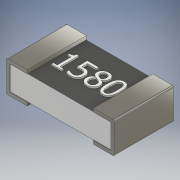
# Autodesk Inventor part: 21-1001
Saved by Autodesk Inventor 2018 (Build 220112000, 112)
## iProperties
Created: 2019-09-21
Part Number: 21-1001
Material: Copper
Document SubType Name: Modeling
Designer: Bradley
Density: 8.94 g/cm^3
Appearance: Smooth - White
Author: Bradley
Autodesk Inventor part; units mm, degrees
ref_plane "YZ Plane" through (0, 0, 0) normal (1, 0, 0) x (0, 1, 0)
ref_plane "XZ Plane" through (0, 0, 0) normal (0, 1, 0) x (-1, 0, 0)
ref_plane "XY Plane" through (0, 0, 0) normal (0, 0, 1) x (1, 0, 0)
sketch "Sketch1" plane through (0, 0, 0) normal (0, 1, 0) x (-1, 0, 0)
  line L0 (0.725, 0.175) -> (-0.725, 0.175)
  line L1 (-0.725, 0.175) -> (-0.725, -0.175)
  line L2 (-0.725, -0.175) -> (0.725, -0.175)
  line L3 (0.725, -0.175) -> (0.725, 0.175)
  line L4 (0.475, 0.175) -> (0.475, 0.225)
  line L5 (0.475, 0.225) -> (0.775, 0.225)
  line L6 (0.775, 0.225) -> (0.775, -0.225)
  line L7 (0.775, -0.225) -> (0.475, -0.225)
  line L8 (0.475, -0.225) -> (0.475, -0.175)
  line L9 (-0.475, 0.175) -> (-0.475, 0.225)
  line L10 (-0.475, 0.225) -> (-0.775, 0.225)
  line L11 (-0.775, 0.225) -> (-0.775, -0.225)
  line L12 (-0.775, -0.225) -> (-0.475, -0.225)
  line L13 (-0.475, -0.175) -> (-0.475, -0.225)
  line L14 (0.475, 0.175) -> (-0.475, 0.175)
  point P0 (0, 0)
  point P1 (0, 0.175)
  point P2 (0.725, 0)
  dimension "d0" = 1.55
  dimension "d1" = 0.05
  dimension "d2" = 0.05
  dimension "d3" = 0.45
  dimension "d4" = 0.3
  constraints: 30 end point, 12 point on line, 7 perpendicular, 3 collinear, 3 midpoint, 2 parallel, 1 horizontal, 1 horizontal alignment, 1 vertical, 1 vertical alignment
  measures "d0" distance between parallel lines of L11 L6
  measures "d1" distance of L7.end L8.end
  measures "d2" distance between parallel lines of L6 L3
  measures "d3" distance of L5.end L6.end
  measures "d4" distance of L6.end L7.end
extrude "Extrusion1" add sketch "Sketch1" along normal mid plane 0.85 contours L0 L4 L5 L6 L7 L8 L2 L3 | L0 L1 L2 L13 L12 L11 L10 L9
extrude "Extrusion2" add sketch "Sketch1" along normal mid plane 0.84 contours L3 L2 L1 L0
sketch "Sketch2" plane through (-0.475, -0.42, 0.175) normal (0, 0, 1) x (1, 0, 0)
  line L0 (0, 0) -> (0, 0.84) projected
  line L1 (0.95, 0) -> (0, 0) projected
  line L2 (0.95, 0) -> (0.95, 0.84) projected
  line L3 (0, 0.84) -> (0.95, 0.84) projected
  line L4 (0, 0.42) -> (0.95, 0.42) construction
  line L5 (0.2166, 0.27) -> (0.0702, 0.27)
  line L6 (0.0702, 0.27) -> (0.0702, 0.3006)
  line L7 (0.0702, 0.3006) -> (0.1247, 0.3006)
  line L8 (0.1247, 0.3006) -> (0.1247, 0.5017)
  line L9 (0.1247, 0.5017) -> (0.0702, 0.5017)
  line L10 (0.0702, 0.5017) -> (0.0702, 0.5292)
  spline S0 degree 2 poles (0.0702, 0.5292) (0.1011, 0.5292) (0.1303, 0.5467) (0.1322, 0.571) knots 0 0 0 1 2 2 2
  line L11 (0.1322, 0.571) -> (0.1633, 0.571)
  line L12 (0.1633, 0.571) -> (0.1633, 0.3006)
  line L13 (0.1633, 0.3006) -> (0.2166, 0.3006)
  line L14 (0.2166, 0.3006) -> (0.2166, 0.27)
  spline S1 degree 2 poles (0.4536, 0.3653) (0.4536, 0.3437) (0.4397, 0.3067) (0.4271, 0.2931) knots 0 0 0 1 2 2 2
  spline S2 degree 2 poles (0.4271, 0.2931) (0.4145, 0.2795) (0.3768, 0.2637) (0.3534, 0.2637) knots 0 0 0 1 2 2 2
  spline S3 degree 2 poles (0.3534, 0.2637) (0.3321, 0.2637) (0.2902, 0.2732) (0.2749, 0.2807) knots 0 0 0 1 2 2 2
  line L15 (0.2749, 0.2807) -> (0.2749, 0.3232)
  line L16 (0.2749, 0.3232) -> (0.2778, 0.3232)
  spline S4 degree 2 poles (0.2778, 0.3232) (0.2825, 0.3198) (0.2997, 0.3111) (0.3102, 0.3072) knots 0 0 0 1 2 2 2
  spline S5 degree 2 poles (0.3102, 0.3072) (0.3221, 0.3031) (0.3418, 0.2984) (0.3542, 0.2984) knots 0 0 0 1 2 2 2
  spline S6 degree 2 poles (0.3542, 0.2984) (0.3663, 0.2984) (0.3892, 0.3072) (0.3974, 0.3167) knots 0 0 0 1 2 2 2
  spline S7 degree 2 poles (0.3974, 0.3167) (0.405, 0.3257) (0.4128, 0.3495) (0.4128, 0.3655) knots 0 0 0 1 2 2 2
  spline S8 degree 2 poles (0.4128, 0.3655) (0.4128, 0.3816) (0.404, 0.402) (0.3957, 0.4088) knots 0 0 0 1 2 2 2
  spline S9 degree 2 poles (0.3957, 0.4088) (0.3872, 0.4164) (0.362, 0.4227) (0.3466, 0.4227) knots 0 0 0 1 2 2 2
  spline S10 degree 2 poles (0.3466, 0.4227) (0.3301, 0.4227) (0.2973, 0.4176) (0.2873, 0.4154) knots 0 0 0 1 2 2 2
  line L17 (0.2873, 0.4154) -> (0.2873, 0.57)
  line L18 (0.2873, 0.57) -> (0.4519, 0.57)
  line L19 (0.4519, 0.57) -> (0.4519, 0.5347)
  line L20 (0.4519, 0.5347) -> (0.326, 0.5347)
  line L21 (0.326, 0.5347) -> (0.326, 0.4548)
  spline S11 degree 2 poles (0.326, 0.4548) (0.3333, 0.4557) (0.3474, 0.4565) (0.3532, 0.4565) knots 0 0 0 1 2 2 2
  spline S12 degree 2 poles (0.3532, 0.4565) (0.3763, 0.4565) (0.4081, 0.4489) (0.4227, 0.4377) knots 0 0 0 1 2 2 2
  spline S13 degree 2 poles (0.4227, 0.4377) (0.4376, 0.4266) (0.4536, 0.3925) (0.4536, 0.3653) knots 0 0 0 1 2 2 2
  spline S14 degree 2 poles (0.5876, 0.2632) (0.5652, 0.2632) (0.5285, 0.2766) (0.5156, 0.289) knots 0 0 0 1 2 2 2
  spline S15 degree 2 poles (0.5156, 0.289) (0.503, 0.3011) (0.4898, 0.3342) (0.4898, 0.3529) knots 0 0 0 1 2 2 2
  spline S16 degree 2 poles (0.4898, 0.3529) (0.4898, 0.3772) (0.5158, 0.4181) (0.5406, 0.4302) knots 0 0 0 1 2 2 2
  line L22 (0.5406, 0.4302) -> (0.5406, 0.4314)
  spline S17 degree 2 poles (0.5406, 0.4314) (0.5185, 0.4443) (0.4971, 0.4749) (0.4971, 0.4978) knots 0 0 0 1 2 2 2
  spline S18 degree 2 poles (0.4971, 0.4978) (0.4971, 0.5316) (0.5482, 0.5768) (0.5876, 0.5768) knots 0 0 0 1 2 2 2
  spline S19 degree 2 poles (0.5876, 0.5768) (0.6284, 0.5768) (0.6778, 0.534) (0.6778, 0.5005) knots 0 0 0 1 2 2 2
  spline S20 degree 2 poles (0.6778, 0.5005) (0.6778, 0.4803) (0.6542, 0.4409) (0.6321, 0.4297) knots 0 0 0 1 2 2 2
  line L23 (0.6321, 0.4297) -> (0.6321, 0.4285)
  spline S21 degree 2 poles (0.6321, 0.4285) (0.6583, 0.4164) (0.6853, 0.3813) (0.6853, 0.3536) knots 0 0 0 1 2 2 2
  spline S22 degree 2 poles (0.6853, 0.3536) (0.6853, 0.3152) (0.6294, 0.2632) (0.5876, 0.2632) knots 0 0 0 1 2 2 2
  spline S23 degree 2 poles (0.644, 0.3497) (0.644, 0.3682) (0.6294, 0.3901) (0.6087, 0.4013) knots 0 0 0 1 2 2 2
  spline S24 degree 2 poles (0.6087, 0.4013) (0.6019, 0.4052) (0.5791, 0.4142) (0.5647, 0.42) knots 0 0 0 1 2 2 2
  spline S25 degree 2 poles (0.5647, 0.42) (0.5482, 0.4091) (0.5304, 0.3765) (0.5304, 0.3558) knots 0 0 0 1 2 2 2
  spline S26 degree 2 poles (0.5304, 0.3558) (0.5304, 0.3286) (0.5632, 0.2931) (0.588, 0.2931) knots 0 0 0 1 2 2 2
  spline S27 degree 2 poles (0.588, 0.2931) (0.6133, 0.2931) (0.644, 0.3235) (0.644, 0.3497) knots 0 0 0 1 2 2 2
  spline S28 degree 2 poles (0.6384, 0.5) (0.6384, 0.5202) (0.6114, 0.5471) (0.5873, 0.5471) knots 0 0 0 1 2 2 2
  spline S29 degree 2 poles (0.5873, 0.5471) (0.5654, 0.5471) (0.5375, 0.5231) (0.5375, 0.5024) knots 0 0 0 1 2 2 2
  spline S30 degree 2 poles (0.5375, 0.5024) (0.5375, 0.4876) (0.5518, 0.4669) (0.5662, 0.4587) knots 0 0 0 1 2 2 2
  spline S31 degree 2 poles (0.5662, 0.4587) (0.5722, 0.4553) (0.598, 0.4433) (0.6085, 0.4399) knots 0 0 0 1 2 2 2
  spline S32 degree 2 poles (0.6085, 0.4399) (0.626, 0.4533) (0.6384, 0.4818) (0.6384, 0.5) knots 0 0 0 1 2 2 2
  spline S33 degree 2 poles (0.9087, 0.42) (0.9087, 0.3393) (0.8618, 0.2637) (0.8129, 0.2637) knots 0 0 0 1 2 2 2
  spline S34 degree 2 poles (0.8129, 0.2637) (0.7633, 0.2637) (0.7169, 0.3407) (0.7169, 0.4198) knots 0 0 0 1 2 2 2
  spline S35 degree 2 poles (0.7169, 0.4198) (0.7169, 0.501) (0.7638, 0.5761) (0.8129, 0.5761) knots 0 0 0 1 2 2 2
  spline S36 degree 2 poles (0.8129, 0.5761) (0.8623, 0.5761) (0.9087, 0.4983) (0.9087, 0.42) knots 0 0 0 1 2 2 2
  spline S37 degree 2 poles (0.8572, 0.3286) (0.863, 0.3434) (0.8679, 0.3891) (0.8679, 0.42) knots 0 0 0 1 2 2 2
  spline S38 degree 2 poles (0.8679, 0.42) (0.8679, 0.4509) (0.863, 0.4963) (0.8569, 0.5117) knots 0 0 0 1 2 2 2
  spline S39 degree 2 poles (0.8569, 0.5117) (0.8509, 0.527) (0.8297, 0.5428) (0.8129, 0.5428) knots 0 0 0 1 2 2 2
  spline S40 degree 2 poles (0.8129, 0.5428) (0.7962, 0.5428) (0.7745, 0.527) (0.7682, 0.5112) knots 0 0 0 1 2 2 2
  spline S41 degree 2 poles (0.7682, 0.5112) (0.7621, 0.4959) (0.7577, 0.4492) (0.7577, 0.4198) knots 0 0 0 1 2 2 2
  spline S42 degree 2 poles (0.7577, 0.4198) (0.7577, 0.3882) (0.7616, 0.3459) (0.7679, 0.3293) knots 0 0 0 1 2 2 2
  spline S43 degree 2 poles (0.7679, 0.3293) (0.7738, 0.3138) (0.7954, 0.297) (0.8129, 0.297) knots 0 0 0 1 2 2 2
  spline S44 degree 2 poles (0.8129, 0.297) (0.8295, 0.297) (0.8511, 0.3128) (0.8572, 0.3286) knots 0 0 0 1 2 2 2
  point P0 (0.475, 0.42)
  constraints: 2 end point, 2 midpoint, 1 horizontal
extrude "Extrusion3" add sketch "Sketch2" along normal blind 0.02 contours L5 L6 L7 L8 L9 L10 S0 L11 L12 L13 L14 | S1 S2 S3 L15 L16 S4 S5 S6 S7 S8 S9 S10 L17 L18 L19 L20 L21 S11 S12 S13 | S14 S15 S16 S17 S18 S19 S20 S21 S22 | S33 S34 S35 S36
fillet "Fillet1" radius 0.02 4 edges at (-0.775, 0, 0.225) (-0.775, 0, -0.225) (0.775, 0, 0.225) (0.775, 0, -0.225)
equation "\"d2\" = d1"
body "Solid1"
